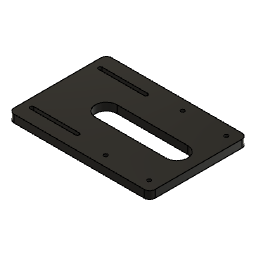
base (Autodesk Fusion 360 design; units mm, degrees)
Autodesk Fusion 360 part; units mm, degrees
sketch "Sketch1" plane through (0, 0, 0) normal (0, 1, 0) x (1, 0, 0)
  line L0 (-65, 45) -> (65, 45)
  line L1 (65, 45) -> (65, -45)
  line L2 (65, -45) -> (-65, -45)
  line L3 (-65, -45) -> (-65, 45)
  circle A0 centre (55, 35.5) radius 1.65
  circle A1 centre (15, 35.5) radius 1.65
  circle A2 centre (55, -35.5) radius 1.65
  circle A3 centre (15, -35.5) radius 1.65
  dimension "d4" = 65
  dimension "d5" = 45
  dimension "d8" = 90
  dimension "d9" = 130
  dimension "d10" = 3.3
  dimension "d12" = 10
  dimension "d13" = 9.5
  dimension "d16" = -40
  dimension "d17" = -71
  constraint horizontal L0
  constraint vertical L1
  constraint horizontal L2
  constraint vertical L3
  measures "d4" distance of origin L3
  measures "d5" distance of origin L2
  measures "d8" distance of L0.end L1.end
  measures "d9" distance of L0.start L0.end
  measures "d10" diameter of A0
  measures "d12" distance of L1 A0.centre
  measures "d13" distance of L0 A0.centre
extrude "Extrude1" add sketch "Sketch1" along normal blind 7
sketch "Sketch2" plane through (0, 7, 0) normal (0, 1, 0) x (-1, 0, 0)
  circle A0 centre (-55, 35.5) radius 1.65
  circle A1 centre (-15, 35.5) radius 1.65
  circle A2 centre (-15, -35.5) radius 1.65
  circle A3 centre (-55, -35.5) radius 1.65
  line L0 (65, 45) -> (-65, 45)
  line L1 (-65, 45) -> (-65, -45)
  line L2 (-65, -45) -> (65, -45)
  line L3 (65, -45) -> (65, 45)
  line L4 (-45, -10) -> (20, -10)
  arc A4 (20, -10) -> (20, 10) centre (20, 0) ccw
  line L5 (20, 10) -> (-45, 10)
  arc A5 (-45, 10) -> (-45, -10) centre (-45, 0) ccw
  line L6 (-45, 0) -> (20, 0) construction
  dimension "d18" = 65
  dimension "d19" = 20
  dimension "d20" = 10
  dimension "d22" = 45
  constraint tangent L4 A4
  constraint tangent A4 L5
  constraint parallel L4 L5
  constraint tangent L5 A5
  constraint tangent L4 A5
  constraint horizontal L6
  measures "d18" distance of A5.centre A4.centre
  measures "d19" distance of L1 A5.centre
  measures "d20" radius of A5
  measures "d22" distance of L0 L6
extrude "Extrude2" cut sketch "Sketch2" against normal up to surface (7 mm away) contours L4 A4 L5 A5
fillet "Fillet1" radius 5 4 edges at (65, 3.5, 45) (-65, 3.5, 45) (-65, 3.5, -45) (65, 3.5, -45)
sketch "Sketch3" plane through (0, 7, 0) normal (0, 1, 0) x (-1, 0, 0)
  arc A0 (-65, -40) -> (-60, -45) centre (-60, -40) ccw
  line L0 (-60, -45) -> (60, -45)
  arc A1 (60, -45) -> (65, -40) centre (60, -40) ccw
  line L1 (65, -40) -> (65, 40)
  arc A2 (65, 40) -> (60, 45) centre (60, 40) ccw
  line L2 (60, 45) -> (-60, 45)
  arc A3 (-60, 45) -> (-65, 40) centre (-60, 40) ccw
  line L3 (-65, 40) -> (-65, -40)
  line L4 (-45, 10) -> (20, 10)
  arc A4 (20, -10) -> (20, 10) centre (20, 0) ccw
  line L5 (20, -10) -> (-45, -10)
  arc A5 (-45, 10) -> (-45, -10) centre (-45, 0) ccw
  circle A6 centre (-55, 35.5) radius 1.65
  circle A7 centre (-15, 35.5) radius 1.65
  circle A8 centre (-15, -35.5) radius 1.65
  circle A9 centre (-55, -35.5) radius 1.65
  line L6 (57, -29.85) -> (15, -29.85)
  arc A10 (15, -29.85) -> (15, -33.15) centre (15, -31.5) ccw
  line L7 (15, -33.15) -> (57, -33.15)
  arc A11 (57, -33.15) -> (57, -29.85) centre (57, -31.5) ccw
  line L8 (57, -31.5) -> (15, -31.5) construction
  line L9 (0, 0) -> (102, 0) construction
  arc A12 (15, 33.15) -> (15, 29.85) centre (15, 31.5) ccw
  line L10 (15, 33.15) -> (57, 33.15)
  line L11 (57, 29.85) -> (15, 29.85)
  arc A13 (57, 29.85) -> (57, 33.15) centre (57, 31.5) ccw
  dimension "d26" = 3.3
  dimension "d27" = 8
  dimension "d28" = 42
  dimension "d30" = 31.5
  constraint tangent L6 A10
  constraint tangent A10 L7
  constraint parallel L6 L7
  constraint tangent L7 A11
  constraint tangent L6 A11
  constraint horizontal L8
  constraint coincident L9.start origin
  constraint horizontal L9
  constraint symmetric L6.start L9 L11.start
  constraint symmetric L6.end L9 A12.end
  constraint symmetric A10.end L9 A12.start
  constraint symmetric L7.end L9 L10.end
  constraint symmetric A10 L9 A12
  constraint symmetric A11 L9 A13
  measures "d26" diameter of A10
  measures "d27" distance of L1 A11.centre
  measures "d28" distance of A11.centre A10.centre
  measures "d30" distance of L8 L9
extrude "Extrude3" cut sketch "Sketch3" against normal up to surface (7 mm away) contours L6 A10 L7 A11 | A12 L10 L11 A13
sketch "Sketch4" plane through (0, 0, 0) normal (0, -1, 0) x (1, 0, 0)
  line L0 (-15, -33.15) -> (-57, -33.15)
  arc A0 (-57, -29.85) -> (-57, -33.15) centre (-57, -31.5) ccw
  line L1 (-57, -29.85) -> (-15, -29.85)
  arc A1 (-15, -33.15) -> (-15, -29.85) centre (-15, -31.5) ccw
  line L2 (-57, 33.15) -> (-15, 33.15)
  arc A2 (-15, 29.85) -> (-15, 33.15) centre (-15, 31.5) ccw
  line L3 (-15, 29.85) -> (-57, 29.85)
  arc A3 (-57, 33.15) -> (-57, 29.85) centre (-57, 31.5) ccw
  line L4 (-20, 10) -> (45, 10)
  arc A4 (45, -10) -> (45, 10) centre (45, 0) ccw
  line L5 (45, -10) -> (-20, -10)
  arc A5 (-20, 10) -> (-20, -10) centre (-20, 0) ccw
  circle A6 centre (55, 35.5) radius 1.65
  circle A7 centre (15, 35.5) radius 1.65
  circle A8 centre (15, -35.5) radius 1.65
  circle A9 centre (55, -35.5) radius 1.65
  arc A10 (60, -45) -> (65, -40) centre (60, -40) ccw
  line L6 (65, -40) -> (65, 40)
  arc A11 (65, 40) -> (60, 45) centre (60, 40) ccw
  line L7 (60, 45) -> (-60, 45)
  arc A12 (-60, 45) -> (-65, 40) centre (-60, 40) ccw
  line L8 (-65, 40) -> (-65, -40)
  arc A13 (-65, -40) -> (-60, -45) centre (-60, -40) ccw
  line L9 (-60, -45) -> (60, -45)
  circle A14 centre (55, 35.5) radius 4
  circle A15 centre (55, -35.5) radius 4
  circle A16 centre (15, 35.5) radius 4
  circle A17 centre (15, -35.5) radius 4
  line L10 (-57, 27.5) -> (-15, 27.5)
  arc A18 (-15, 27.5) -> (-15, 35.5) centre (-15, 31.5) ccw
  line L11 (-15, 35.5) -> (-57, 35.5)
  arc A19 (-57, 35.5) -> (-57, 27.5) centre (-57, 31.5) ccw
  line L12 (-57, 31.5) -> (-15, 31.5) construction
  line L13 (-57, -35.5) -> (-15, -35.5)
  arc A20 (-15, -35.5) -> (-15, -27.5) centre (-15, -31.5) ccw
  line L14 (-15, -27.5) -> (-57, -27.5)
  arc A21 (-57, -27.5) -> (-57, -35.5) centre (-57, -31.5) ccw
  line L15 (-57, -31.5) -> (-15, -31.5) construction
  dimension "d33" = 8
  dimension "d34" = 8
  dimension "d35" = 8
  dimension "d36" = 8
  dimension "d37" = 8
  dimension "d38" = 8
  constraint concentric A6 A14
  constraint concentric A9 A15
  constraint concentric A7 A16
  constraint concentric A8 A17
  constraint tangent L10 A18
  constraint tangent A18 L11
  constraint parallel L10 L11
  constraint tangent L11 A19
  constraint tangent L10 A19
  constraint coincident A2.centre A18.centre
  constraint parallel L3 L12
  constraint coincident A3.centre A19.centre
  constraint tangent L13 A20
  constraint tangent A20 L14
  constraint parallel L13 L14
  constraint tangent L14 A21
  constraint tangent L13 A21
  constraint coincident A1.centre A20.centre
  constraint parallel L0 L15
  constraint coincident A0.centre A21.centre
  measures "d33" diameter of A14
  measures "d34" diameter of A15
  measures "d35" diameter of A16
  measures "d36" diameter of A17
  measures "d37" diameter of A18
  measures "d38" diameter of A20
extrude "Extrude4" cut sketch "Sketch4" against normal blind 3 contours A14 | A15 | A16 | A17 | L10 A18 L11 A19 | L13 A20 L14 A21
equation "length = 130 mm"
equation "width = 90 mm"
equation "thickness = 7 mm"
equation "d4 = length / 2"
equation "d5 = width / 2"
equation "d6 = thickness"
equation "d8 = width"
equation "d9 = length"
equation "d10 = d11"
equation "d11 = 3.3 mm"
equation "d13 = ( width - 71 mm ) / 2"
equation "d22 = width / 2"
equation "d30 = ( 63 / 2 ) * 1 mm"
